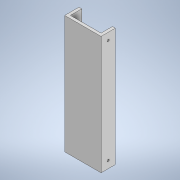
# Autodesk Inventor part: board-1-new
Saved by Autodesk Inventor 2020 (Build 240168000, 168)
## iProperties
Created: 2020-12-14
Part Number: board-1-new
Material: Типовые
Document SubType Name: Modeling
Designer: Alkhimov
Density: 1 g/cm^3
Appearance: По умолчанию
Author: Alkhimov
Autodesk Inventor part; units mm, degrees
ref_plane "YZ Plane" through (0, 0, 0) normal (1, 0, 0) x (0, 1, 0)
ref_plane "XZ Plane" through (0, 0, 0) normal (0, 1, 0) x (-1, 0, 0)
ref_plane "XY Plane" through (0, 0, 0) normal (0, 0, 1) x (1, 0, 0)
sketch "Эскиз1" plane through (0, 0, 0) normal (0, 1, 0) x (-1, 0, 0)
  line L0 (12.75, -5) -> (-12.75, -5)
  line L1 (-12.75, -5) -> (-12.75, 5)
  line L2 (-12.75, 5) -> (12.75, 5)
  line L3 (12.75, 5) -> (12.75, -5)
  line L4 (-12.75, -5) -> (12.75, 5) construction
  line L5 (12.75, -5) -> (-12.75, 5) construction
  line L6 (-10.75, -3) -> (10.75, -3)
  line L7 (10.75, -3) -> (10.75, 3)
  line L8 (10.75, 3) -> (-10.75, 3)
  line L9 (-10.75, 3) -> (-10.75, -3)
  point P0 (0, 0)
  point P1 (0, 0)
  dimension "d0" = 25.5
  dimension "d1" = 10
  dimension "d2" = 2
  constraints: 20 end point, 4 parallel, 2 perpendicular, 1 coincident, 1 horizontal, 1 midpoint, 3 other
  measures "d0" distance of L0.start L0.end
  measures "d1" distance of L0.end L1.end
  measures "d2" distance between parallel lines of L0 L6
extrude "Выдавливание1" add sketch "Эскиз1" along normal blind 82.9
sketch "Эскиз3" plane through (12.75, 0, -5) normal (0, 0, -1) x (-1, 0, 0)
  line L0 (0, 0) -> (0, 82.9) projected
  line L1 (25.5, 0) -> (25.5, 82.9) projected
  line L2 (25.5, 0) -> (25.5, 82.9) projected
  line L3 (0, 0) -> (0, 82.9) projected
  line L4 (0, 82.9) -> (25.5, 82.9) projected
  arc A0 (2, 72.9) -> (23.5, 72.9) centre (12.75, 72.9) ccw
  line L5 (23.5, 0) -> (23.5, 82.9) projected
  line L6 (2, 0) -> (2, 82.9) projected
  line L7 (23.5, 0) -> (23.5, 82.9) projected
  line L8 (23.5, 72.9) -> (23.5, 82.9)
  line L9 (23.5, 82.9) -> (2, 82.9)
  line L10 (2, 72.9) -> (2, 82.9)
  point P0 (12.75, 0)
  dimension "d10" = 10
  constraints: 6 end point, 3 tangent, 2 collinear, 2 point on circle, 2 point on line, 1 centre point, 1 perpendicular
  measures "d10" distance from line of L4 A0.centre
extrude "Выдавливание3" cut sketch "Эскиз3" against normal up to surface (2 mm away)
sketch "Эскиз2" plane through (12.75, 0, 5) normal (1, 0, 0) x (0, 0, -1)
  line L0 (0, 82.9) -> (10, 82.9) construction
  line L1 (10, 82.9) -> (0, 72.9) construction
  line L2 (0, 0) -> (0, 82.9) construction
  line L3 (0, 82.9) -> (10, 72.9) construction
  line L4 (10, 0) -> (10, 82.9) construction
  line L5 (10, 0) -> (0, 10) construction
  line L6 (0, 0) -> (10, 10) construction
  circle A0 centre (5, 77.9) radius 0.5
  circle A1 centre (5, 5) radius 0.5
  point P0 (5, 0)
  dimension "d5" = 1
  dimension "d6" = 1
  constraints: 8 end point, 4 perpendicular, 4 point on line, 2 centre point, 2 midpoint
  measures "d5" diameter of A0
  measures "d6" diameter of A1
hole "Отверстие1" at (12.75, 77.9, 0) at (12.75, 5, 0) direction (-1, 0, 0) diameter 1 depth 2 countersink diameter 1.5 countersink angle 90
mirror "Зеркальное отражение1" about plane through (0, 0, 0) normal (1, 0, 0) of "Отверстие1"
